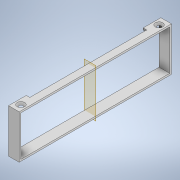
# Autodesk Inventor part: front ring part
Saved by Autodesk Inventor 2020.1 (Build 241239000, 239)
## iProperties
Created: 2019-08-22
Part Number: front ring part
Material: Generic
Document SubType Name: Modeling
Designer: jjsch
Density: 1 g/cm^3
Appearance: Default
Author: jjsch
Autodesk Inventor part; units mm, degrees
ref_plane "YZ Plane" through (0, 0, 0) normal (1, 0, 0) x (0, 1, 0)
ref_plane "XZ Plane" through (0, 0, 0) normal (0, 1, 0) x (-1, 0, 0)
ref_plane "XY Plane" through (0, 0, 0) normal (0, 0, 1) x (1, 0, 0)
sketch "Sketch1" plane through (0, 0, 0) normal (1, 0, 0) x (0, 1, 0)
  line L0 (5.2806, 87.403) -> (-40.1194, 87.403)
  line L1 (-40.1194, 87.403) -> (-40.1194, -80.597)
  line L2 (-40.1194, -80.597) -> (5.2806, -80.597)
  line L3 (5.2806, -80.597) -> (5.2806, 87.403)
  line L4 (7.2806, 89.403) -> (-42.1194, 89.403)
  line L5 (-42.1194, 89.403) -> (-42.1194, -82.597)
  line L6 (-42.1194, -82.597) -> (7.2806, -82.597)
  line L7 (7.2806, -82.597) -> (7.2806, 89.403)
  point P0 (0, 0)
  dimension "d0" = 168
  dimension "d1" = 45.4
  dimension "d2" = 2
  constraints: 16 end point, 4 parallel, 2 perpendicular, 1 horizontal, 3 other
  measures "d0" distance of L0.end L1.end
  measures "d1" distance of L0.start L0.end
  measures "d2" distance between parallel lines of L3 L7
extrude "Extrusion1" add sketch "Sketch1" along normal blind 12
sketch "Sketch2" plane through (0, 7.2806, 89.403) normal (0, 1, 0) x (1, 0, 0)
  line L0 (12, 172) -> (12, 0) projected
  line L1 (0, 0) -> (12, 0) projected
  point P0 (0, 89.403)
  point P1 (6, 8)
  dimension "d5" = 6
  dimension "d6" = 8
  measures "d5" distance from line of L0 point (6, 8)
  measures "d6" distance from line of L1 point (6, 8)
hole "Hole1" at (6, 7.2806, 81.403) direction (0, -1, 0) diameter 4 depth 10 tip angle 118 countersink diameter 8.4 countersink angle 90
ref_plane "Work Plane1" through (0, -42.1194, 3.403) normal (0, 0, 1) x (1, 0, 0)
mirror "Mirror1" about plane through (0, -42.1194, 3.403) normal (0, 0, 1) of "Hole1"
sketch "Sketch3" plane through (0, 7.2806, 89.403) normal (0, 1, 0) x (1, 0, 0)
  line L0 (0, 0) -> (0, 172) projected
  line L1 (0, 20) -> (4, 20)
  line L2 (4, 20) -> (4, 152)
  line L3 (4, 152) -> (0, 152)
  line L4 (0, 152) -> (0, 20)
  line L5 (0, 0) -> (12, 0) projected
  line L6 (0, 172) -> (12, 172) projected
  point P0 (0, 89.403)
  point P1 (0, 152)
  dimension "d14" = 20
  dimension "d15" = 20
  dimension "d16" = 4
  constraints: 8 end point, 2 parallel, 1 horizontal, 1 perpendicular, 1 point on line
  measures "d14" distance between parallel lines of L5 L1
  measures "d15" distance between parallel lines of L6 L3
  measures "d16" distance between parallel lines of L0 L2
extrude "Extrusion2" cut sketch "Sketch3" against normal blind 10
body "Solid1"
